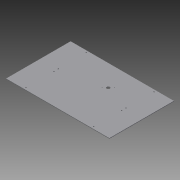
# Autodesk Inventor part: lift plate
Saved by Autodesk Inventor 2015 SP1 (Build 190203100, 203)
## iProperties
Created: 2015-01-13
Part Number: lift plate
Material: Generic
Document SubType Name: Modeling
Designer: Jarod
Density: 1 g/cm^3
Appearance: Default
Author: Jarod
Autodesk Inventor part; units mm, degrees
ref_plane "YZ Plane" through (0, 0, 0) normal (1, 0, 0) x (0, 1, 0)
ref_plane "XZ Plane" through (0, 0, 0) normal (0, 1, 0) x (-1, 0, 0)
ref_plane "XY Plane" through (0, 0, 0) normal (0, 0, 1) x (1, 0, 0)
sketch "Sketch1" plane through (0, 0, 0) normal (0, 1, 0) x (-1, 0, 0)
  line L0 (0, 0) -> (660.4, 0)
  line L1 (660.4, 0) -> (660.4, 406.4)
  line L2 (660.4, 406.4) -> (0, 406.4)
  line L3 (0, 406.4) -> (0, 0)
  dimension "d0" = 660.4
  dimension "d1" = 406.4
  constraints: 8 end point, 2 parallel, 1 horizontal, 1 perpendicular
  measures "d0" distance of L2.end L1.end
  measures "d1" distance of L1.end L0.end
extrude "Extrusion1" add sketch "Sketch1" along normal blind 3.175
sketch "Sketch2" plane through (0, 3.175, 0) normal (0, 1, 0) x (1, 0, 0)
  line L0 (0, 0) -> (-660.4, 0) projected
  line L1 (-660.4, 0) -> (-660.4, -406.4) projected
  line L2 (-660.4, -406.4) -> (0, -406.4) projected
  line L3 (0, -406.4) -> (0, 0) projected
  point P0 (-127, -381)
  point P1 (-533.4, -381)
  point P2 (-533.4, -25.4)
  point P3 (-127, -25.4)
  dimension "d4" = 127
  dimension "d5" = 127
  dimension "d6" = 127
  dimension "d7" = 127
  dimension "d8" = 25.4
  dimension "d9" = 25.4
  dimension "d10" = 25.4
  dimension "d11" = 25.4
  measures "d4" distance from line of L3 point (-127, -381)
  measures "d5" distance from line of point (-127, -25.4) L3
  measures "d6" distance from line of L1 point (-533.4, -381)
  measures "d7" distance from line of L1 point (-533.4, -25.4)
  measures "d8" distance from line of L0 point (-533.4, -25.4)
  measures "d9" distance from line of L2 point (-533.4, -381)
  measures "d10" distance from line of L2 point (-127, -381)
  measures "d11" distance from line of L0 point (-127, -25.4)
hole "Hole1" at (-127, 3.175, 381) at (-533.4, 3.175, 381) at (-533.4, 3.175, 25.4) at (-127, 3.175, 25.4) direction (0, -1, 0) diameter 6.35 end through all
sketch "Sketch3" plane through (0, 3.175, 0) normal (0, 1, 0) x (1, 0, 0)
  circle A0 centre (-533.4, -25.4) radius 3.175 projected
  circle A1 centre (-127, -381) radius 3.175 projected
  circle A2 centre (-533.4, -381) radius 3.175 projected
  circle A3 centre (-127, -25.4) radius 3.175 projected
  line L0 (0, 0) -> (-660.4, 0) projected
  line L1 (-660.4, 0) -> (-660.4, -406.4) projected
  line L2 (-660.4, -406.4) -> (0, -406.4) projected
  line L3 (0, -406.4) -> (0, 0) projected
  point P0 (-127, -228.6)
  point P1 (-127, -177.8)
  point P2 (-533.4, -177.8)
  point P3 (-533.4, -228.6)
  dimension "d19" = 177.8
  dimension "d20" = 177.8
  dimension "d21" = 177.8
  dimension "d22" = 177.8
  dimension "d23" = 127
  dimension "d24" = 127
  dimension "d25" = 127
  dimension "d26" = 127
  measures "d19" distance from line of L2 point (-127, -228.6)
  measures "d20" distance from line of L0 point (-127, -177.8)
  measures "d21" distance from line of L2 point (-533.4, -228.6)
  measures "d22" distance from line of L0 point (-533.4, -177.8)
  measures "d23" distance from line of L1 point (-533.4, -228.6)
  measures "d24" distance from line of L1 point (-533.4, -177.8)
  measures "d25" distance from line of point (-127, -177.8) L3
  measures "d26" distance from line of L3 point (-127, -228.6)
hole "Hole2" at (-127, 3.175, 228.6) at (-127, 3.175, 177.8) at (-533.4, 3.175, 177.8) at (-533.4, 3.175, 228.6) direction (0, -1, 0) diameter 6.35 end through all
sketch "Sketch4" plane through (0, 3.175, 0) normal (0, 1, 0) x (1, 0, 0)
  circle A0 centre (-533.4, -177.8) radius 3.175 projected
  circle A1 centre (-127, -228.6) radius 3.175 projected
  circle A2 centre (-127, -177.8) radius 3.175 projected
  circle A3 centre (-533.4, -228.6) radius 3.175 projected
  circle A4 centre (-533.4, -25.4) radius 3.175 projected
  circle A5 centre (-127, -381) radius 3.175 projected
  circle A6 centre (-533.4, -381) radius 3.175 projected
  circle A7 centre (-127, -25.4) radius 3.175 projected
  line L0 (0, 0) -> (-660.4, 0) projected
  line L1 (-660.4, 0) -> (-660.4, -406.4) projected
  line L2 (-660.4, -406.4) -> (0, -406.4) projected
  line L3 (0, -406.4) -> (0, 0) projected
  circle A8 centre (-330.2, -127) radius 9.525
  line L4 (-330.2, -127) -> (-348.1605, -144.9605) construction
  line L5 (-330.2, -127) -> (-304.8, -127) construction
  line L6 (-330.2, -127) -> (-312.2395, -109.0395) construction
  line L7 (-330.2, -127) -> (-304.8, -127) construction
  circle A9 centre (-348.1605, -144.9605) radius 1.9844
  circle A10 centre (-312.2395, -109.0395) radius 1.9844
  dimension "d34" = 19.05
  dimension "d35" = 127
  dimension "d36" = 330.2
  dimension "d37" = 25.4
  dimension "d38" = 135
  dimension "d39" = 25.4
  dimension "d40" = 45
  dimension "d41" = 3.9688
  dimension "d42" = 3.9688
  constraints: 8 end point, 3 centre point, 2 coincident, 2 equal length, 2 horizontal
  measures "d34" diameter of A8
  measures "d35" distance from line of L0 L4.start
  measures "d36" distance from line of L4.start L3
  measures "d37" distance of L4.start L4.end
  measures "d38" angle of L4 L5
  measures "d39" distance of L4.start L6.end
  measures "d40" angle of L7 L6
  measures "d41" diameter of A9
  measures "d42" diameter of A10
extrude "Extrusion2" cut sketch "Sketch4" against normal blind 3.175 contours A8 | A9 | A10
body "Solid1"
